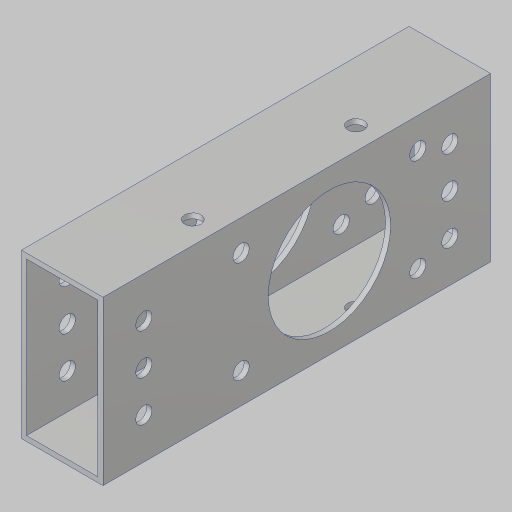
# Autodesk Inventor part: GP5-001
Saved by Autodesk Inventor 2023.5 (Build 275446000, 446)
## iProperties
RuleStatus: InUse
Created: 2025-01-28
Part Number: GP5-001
Material: Aluminum 6061
Document SubType Name: Modeling
Designer: slick
Mass: 304.185 g
Surface Area: 718.547 cm^2
Volume: 112.661 cm^3
Density: 2.7 g/cm^3
Appearance: Aluminum - Flat
AfterDocNew0: SHOW
AfterDocOpen0: SHOW
Author: slick
Autodesk Inventor part; units mm, degrees
ref_plane "YZ Plane" through (0, 0, 0) normal (1, 0, 0) x (0, 1, 0)
ref_plane "XZ Plane" through (0, 0, 0) normal (0, 1, 0) x (-1, 0, 0)
ref_plane "XY Plane" through (0, 0, 0) normal (0, 0, 1) x (1, 0, 0)
sketch "Sketch1" plane through (0, 0, 0) normal (0, 0, 1) x (1, 0, 0)
  line L0 (-12.7, -25.4) -> (12.7, -25.4)
  line L1 (12.7, -25.4) -> (12.7, 25.4)
  line L2 (12.7, 25.4) -> (-12.7, 25.4)
  line L3 (-12.7, 25.4) -> (-12.7, -25.4)
  line L4 (-12.7, -25.4) -> (12.7, 25.4) construction
  line L5 (12.7, -25.4) -> (-12.7, 25.4) construction
  line L6 (-11.1125, 23.8125) -> (11.1125, 23.8125)
  line L7 (11.1125, 23.8125) -> (11.1125, -23.8125)
  line L8 (11.1125, -23.8125) -> (-11.1125, -23.8125)
  line L9 (-11.1125, -23.8125) -> (-11.1125, 23.8125)
  point P0 (0, 0)
  dimension "width" = 25.4
  dimension "height" = 50.8
  dimension "thickness" = 1.5875
  constraints: 20 end point, 4 parallel, 2 midpoint, 2 perpendicular, 1 horizontal, 3 other
  measures "width" distance of L2.end L1.end
  measures "height" distance of L1.end L0.end
  measures "thickness" distance between parallel lines of L2 L6
extrude "Extrusion1" add sketch "Sketch1" along normal mid plane 120.65
sketch "Sketch2" plane through (-12.7, -25.4, 60.325) normal (-1, 0, 0) x (0, 0, 1)
  circle A0 centre (-70.485, 25.4) radius 31.75 construction
  line L0 (-120.65, 0) -> (-120.65, 50.8) projected
  line L1 (-60.325, 50.8) -> (-60.325, 0) construction
  line L2 (0, 0) -> (-120.65, 0) construction
  line L3 (-120.65, 50.8) -> (0, 50.8) construction
  circle A1 centre (-70.485, 25.4) radius 19.05
  point P0 (-107.95, 38.1)
  point P1 (-107.95, 25.4)
  point P2 (-107.95, 12.7)
  point P3 (-12.7, 38.1)
  point P4 (-12.7, 25.4)
  point P5 (-12.7, 12.7)
  point P6 (-70.485, 57.15)
  point P7 (-60.325, 25.4)
  point P8 (-97.9813, 41.275)
  point P9 (-97.9813, 9.525)
  point P10 (-70.485, -6.35)
  point P11 (-42.9887, 9.525)
  point P12 (-42.9887, 41.275)
  dimension "d5" = 63.5
  dimension "d17" = 12.7
  dimension "d18" = 12.7
  dimension "d19" = 12.7
  dimension "d23" = 10.16
  dimension "d26" = 360
  dimension "d28" = 38.1
  constraints: 4 midpoint, 4 vertical alignment, 3 symmetric about line, 2 end point, 2 horizontal alignment, 1 centre point, 1 coincident, 9 other
  measures "d17" distance of point (-107.95, 38.1) point (-107.95, 25.4)
  measures "d18" distance of point (-107.95, 12.7) point (-107.95, 25.4)
  measures "d19" distance from line of L0 point (-107.95, 38.1)
  measures "d23" horizontal distance of point (-60.325, 50.8) point (-70.485, 25.4)
  measures "d28" diameter of A1
hole "Hole1" at (-12.7, 12.7, -47.625) at (-12.7, 0, -47.625) at (-12.7, -12.7, -47.625) at (-12.7, -12.7, 47.625) at (-12.7, 0, 47.625) at (-12.7, 12.7, 47.625) at (-12.7, 15.875, 17.3363) at (-12.7, -15.875, 17.3363) at (-12.7, -15.875, -37.6563) at (-12.7, 15.875, -37.6563) direction (1, 0, 0) diameter 5.1054 end through all clearance for "Flat Head Machine Screw (82)" size "#10" standard "Ansi Unified Screw Threads"
extrude "Extrusion3" cut sketch "Sketch2" against normal through all
sketch "Sketch4" plane through (-12.7, 25.4, 60.325) normal (0, 1, 0) x (1, 0, 0)
  line L0 (18.415, 34.925) -> (18.415, 85.725) construction
  line L1 (25.4, 0) -> (0, 0) construction
  line L2 (0, 120.65) -> (0, 0) construction
  point P0 (18.415, 60.325)
  point P1 (12.7, 0)
  point P2 (0, 60.325)
  dimension "d41" = 50.8
  dimension "d42" = 18.415
  constraints: 3 midpoint, 2 coincident, 2 end point, 1 horizontal alignment, 1 vertical
  measures "d41" distance of L0.start L0.end
  measures "d42" distance between parallel lines of L2 L0
hole "Hole2" at (5.715, 25.4, -25.4) at (5.715, 25.4, 25.4) direction (0, -1, 0) diameter 5.1054 end through all clearance for "Flat Head Machine Screw (82)" size "#10" standard "Ansi Unified Screw Threads"
body "Solid1"
